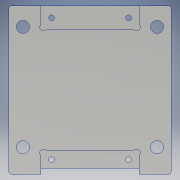
# Autodesk Inventor part: Part2
Saved by Autodesk Inventor 2018 (Build 220112000, 112)
## iProperties
Created: 2018-02-06
Part Number: Part2
Material: Aluminum 6061
Document SubType Name: Modeling
Designer: P136265
Density: 2.7 g/cm^3
Appearance: Aluminum - Flat
Author: P136265
Autodesk Inventor part; units mm, degrees
ref_plane "YZ Plane" through (0, 0, 0) normal (1, 0, 0) x (0, 1, 0)
ref_plane "XZ Plane" through (0, 0, 0) normal (0, 1, 0) x (-1, 0, 0)
ref_plane "XY Plane" through (0, 0, 0) normal (0, 0, 1) x (1, 0, 0)
sketch "Sketch1" plane through (0, 0, 0) normal (0, 1, 0) x (-1, 0, 0)
  line L0 (67.5, -70) -> (-67.5, -70)
  line L1 (-67.5, -70) -> (-67.5, 70)
  line L2 (-67.5, 70) -> (67.5, 70)
  line L3 (67.5, 70) -> (67.5, -70)
  line L4 (67.5, -70) -> (-67.5, 70) construction
  line L5 (-67.5, -70) -> (67.5, 70) construction
  circle A0 centre (-55.75, -52.5) radius 5.5
  circle A1 centre (55.75, -52.5) radius 5.5
  circle A2 centre (55.75, 47.5) radius 5.5
  circle A3 centre (-55.75, 47.5) radius 5.5
  line L6 (55.75, -52.5) -> (-55.75, -52.5) construction
  line L7 (55.75, 47.5) -> (-55.75, 47.5) construction
  line L8 (0, -70) -> (0, -52.5) construction
  line L9 (0, -52.5) -> (0, 0) construction
  line L10 (0, 0) -> (0, 47.5) construction
  line L11 (0, 70) -> (0, 47.5) construction
  point P0 (0, 0)
  point P1 (0, 0)
  point P2 (0, 0)
  dimension "d0" = 135
  dimension "d1" = 140
  dimension "d2" = 11
  dimension "d4" = 11
  dimension "d5" = 11
  dimension "d6" = 11
  dimension "d7" = 111.5
  dimension "d9" = 100
  dimension "d27" = 22.5
  constraints: 24 end point, 8 midpoint, 4 centre point, 3 horizontal, 2 collinear, 2 parallel, 2 vertical alignment, 1 coincident, 1 perpendicular
  measures "d0" distance of L1.end L2.end
  measures "d1" distance of L0.end L1.end
  measures "d2" diameter of A0
  measures "d4" diameter of A1
  measures "d5" diameter of A2
  measures "d6" diameter of A3
  measures "d7" distance of L6.end L6.start
  measures "d9" distance of L7.start L6.start
  measures "d27" distance from line of L2 L7.start
extrude "Extrusion1" add sketch "Sketch1" along normal blind 5
sketch "Sketch3" plane through (0, 5, 0) normal (0, 1, 0) x (1, 0, 0)
  circle A0 centre (55.75, -47.5) radius 5.5 construction
  circle A1 centre (-55.75, -47.5) radius 5.5 construction
  circle A2 centre (-55.75, 52.5) radius 5.5 construction
  circle A3 centre (55.75, 52.5) radius 5.5 construction
  line L0 (67.5, 70) -> (-67.5, 70) construction
  line L1 (-67.5, 70) -> (-67.5, -70) construction
  line L2 (-67.5, -70) -> (67.5, -70) construction
  line L3 (67.5, -70) -> (67.5, 70) construction
  line L4 (-41, -70) -> (41, -70)
  line L5 (-36.7574, -50) -> (36.7574, -50)
  line L6 (-41, -54.2426) -> (-41, -70)
  line L7 (41, -54.2426) -> (41, -70)
  line L8 (-67.5, -70) -> (67.5, -70) construction
  line L9 (-67.5, 70) -> (-67.5, -70) construction
  line L10 (-67.5, 0) -> (67.5, 0) construction
  line L11 (67.5, -70) -> (67.5, 70) construction
  arc A4 (-36.7574, -50) -> (-41, -54.2426) centre (-38.8787, -52.1213) ccw
  line L12 (-41, -50) -> (-38.8787, -52.1213) construction
  line L13 (0, -50) -> (0, -70) construction
  arc A5 (41, -54.2426) -> (36.7574, -50) centre (38.8787, -52.1213) ccw
  line L14 (-41, 70) -> (41, 70)
  line L15 (-36.7574, 50) -> (36.7574, 50)
  line L16 (-41, 54.2426) -> (-41, 70)
  line L17 (41, 54.2426) -> (41, 70)
  arc A6 (-41, 54.2426) -> (-36.7574, 50) centre (-38.8787, 52.1213) ccw
  line L18 (-41, 50) -> (-38.8787, 52.1213) construction
  line L19 (0, 50) -> (0, 70) construction
  arc A7 (36.7574, 50) -> (41, 54.2426) centre (38.8787, 52.1213) ccw
  circle A8 centre (55.75, -47.5) radius 5.5 projected
  circle A9 centre (-55.75, -47.5) radius 5.5 projected
  circle A10 centre (-55.75, 52.5) radius 5.5 projected
  circle A11 centre (55.75, 52.5) radius 5.5 projected
  line L20 (-67.5, 70) -> (67.5, 70) projected
  line L21 (67.5, 70) -> (67.5, -70) projected
  line L22 (67.5, -70) -> (-67.5, -70) projected
  line L23 (-67.5, -70) -> (-67.5, 70) projected
  point P0 (0, 0)
  point P1 (41, -50)
  point P2 (0, -70)
  point P3 (0, -70)
  point P4 (41, 50)
  point P5 (0, 70)
  point P6 (0, 70)
  dimension "d19" = 82
  dimension "d20" = 20
  dimension "d67" = 6
  dimension "d68" = 45
  dimension "d70" = 73.5147
  dimension "d71" = 15.7574
  dimension "d72" = 120
  dimension "d73" = 26.5
  constraints: 26 end point, 18 symmetric about line, 10 point on circle, 7 midpoint, 4 centre point, 4 coincident, 2 parallel, 2 perpendicular, 1 horizontal, 3 other
  measures "d19" distance of L4.start L4.end
  measures "d20" distance between parallel lines of L4 L5
  measures "d67" diameter of A4
  measures "d68" angle of L12 L6
  measures "d70" distance of L5.end L5.start
  measures "d71" distance of L4.end L7.start
  measures "d72" distance from line of point (41, -50) L0
  measures "d73" distance from line of point (41, -50) L11
extrude "Extrusion3" cut sketch "Sketch3" against normal blind 1 contours L6 A4 L5 A5 L7 L4 | L14 L17 A7 L15 A6 L16
fillet "Fillet1" radius 2 4 edges at (67.5, 2.5, 70) (-67.5, 2.5, 70) (-67.5, 2.5, -70) (67.5, 2.5, -70)
sketch "Sketch4" plane through (0, 0, 0) normal (0, -1, 0) x (1, 0, 0)
  arc A0 (65.5, -70) -> (67.5, -68) centre (65.5, -68) ccw construction
  line L0 (67.5, -68) -> (67.5, 68) construction
  arc A1 (67.5, 68) -> (65.5, 70) centre (65.5, 68) ccw construction
  line L1 (65.5, 70) -> (-65.5, 70) construction
  arc A2 (-65.5, 70) -> (-67.5, 68) centre (-65.5, 68) ccw construction
  line L2 (-67.5, 68) -> (-67.5, -68) construction
  arc A3 (-67.5, -68) -> (-65.5, -70) centre (-65.5, -68) ccw construction
  line L3 (-65.5, -70) -> (65.5, -70) construction
  circle A4 centre (55.75, 47.5) radius 5.5 construction
  circle A5 centre (-55.75, 47.5) radius 5.5 construction
  circle A6 centre (-55.75, -52.5) radius 5.5 construction
  circle A7 centre (55.75, -52.5) radius 5.5 construction
  line L4 (-41, 70) -> (41, 70)
  line L5 (-41, 65) -> (41, 65)
  line L6 (-41, 70) -> (-41, 65)
  line L7 (41, 70) -> (41, 65)
  line L8 (65.5, 70) -> (-65.5, 70) construction
  point P0 (0, 0)
  point P1 (0, 70)
  point P2 (0, 70)
  point P3 (0, 70)
  dimension "d30" = 82
  dimension "d31" = 5
  constraints: 8 end point, 3 midpoint, 2 coincident, 2 parallel, 1 horizontal, 1 vertical
  measures "d30" distance of L4.start L4.end
  measures "d31" distance between parallel lines of L4 L5
extrude "Extrusion4" cut sketch "Sketch4" against normal up to next
sketch "Sketch7" plane through (0, 0, 0) normal (0, -1, 0) x (1, 0, 0)
  arc A0 (67.5, 68) -> (65.5, 70) centre (65.5, 68) ccw projected
  line L0 (67.5, 68) -> (40.95, 68) construction
  line L1 (41, 70) -> (65.5, 70) projected
  line L2 (40.95, 68) -> (41, 70)
  line L3 (41, 70) -> (32, 70) construction
  line L4 (32, 70) -> (32, 58) construction
  circle A1 centre (32, 58) radius 3
  line L5 (32, 58) -> (-32, 58) construction
  circle A2 centre (-32, 58) radius 3
  line L6 (-67.5, -70) -> (-40.95, -70) construction
  line L7 (-65.5, -70) -> (65.5, -70) projected
  line L8 (-40.95, -70) -> (-31.95, -70) construction
  line L9 (-31.95, -70) -> (-31.95, -60) construction
  line L10 (-31.95, -60) -> (32.05, -60) construction
  circle A3 centre (-31.95, -60) radius 3
  circle A4 centre (32.05, -60) radius 3
  point P0 (0, 0)
  dimension "d78" = 26.55
  dimension "d79" = 9
  dimension "d80" = 12
  dimension "d81" = 6
  dimension "d82" = 64
  dimension "d84" = 6
  dimension "d85" = 26.55
  dimension "d86" = 9
  dimension "d87" = 10
  dimension "d88" = 64
  dimension "d89" = 6
  dimension "d90" = 6
  dimension "d92" = 63.95
  constraints: 18 end point, 4 centre point, 4 coincident, 3 horizontal, 2 parallel, 2 perpendicular, 2 point on line
  measures "d78" distance of L0.start L0.end
  measures "d79" distance of L1.start L3.end
  measures "d80" distance of L3.end L4.end
  measures "d81" diameter of A1
  measures "d82" distance of L5.start L5.end
  measures "d84" diameter of A2
  measures "d85" distance of L6.start L6.end
  measures "d86" distance of L6.end L8.end
  measures "d87" distance of L8.end L9.end
  measures "d88" distance of L9.end L10.end
  measures "d89" diameter of A3
  measures "d90" diameter of A4
  measures "d92" distance between parallel lines of L9 L4
hole "Hole3" at (32, 0, 58) at (-32, 0, 58) at (-31.95, 0, -60) at (32.05, 0, -60) direction (0, 1, 0) diameter 5 end through all countersink diameter 12 countersink angle 90
body "Solid1"
